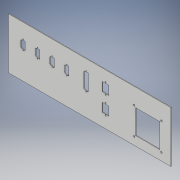
# Autodesk Inventor part: PDU_chassis
Saved by Autodesk Inventor 2017 (Build 210142000, 142)
## iProperties
Created: 2017-02-13
Part Number: PDU_chassis
Material: Generic
Document SubType Name: Modeling
Designer: Zara
Density: 1 g/cm^3
Appearance: Default
Author: Zara
Autodesk Inventor part; units mm, degrees
ref_plane "YZ Plane" through (0, 0, 0) normal (1, 0, 0) x (0, 1, 0)
ref_plane "XZ Plane" through (0, 0, 0) normal (0, 1, 0) x (-1, 0, 0)
ref_plane "XY Plane" through (0, 0, 0) normal (0, 0, 1) x (1, 0, 0)
sketch "Sketch1" plane through (0, 0, 0) normal (0, 0, 1) x (1, 0, 0)
  line L0 (-212.471, -66.7512) -> (212.471, -66.7512)
  line L1 (212.471, -66.7512) -> (212.471, 66.7512)
  line L2 (212.471, 66.7512) -> (-212.471, 66.7512)
  line L3 (-212.471, 66.7512) -> (-212.471, -66.7512)
  line L4 (-212.471, -66.7512) -> (212.471, 66.7512) construction
  line L5 (212.471, -66.7512) -> (-212.471, 66.7512) construction
  point P0 (0, 0)
  dimension "d0" = 424.942
  dimension "d1" = 133.5024
  constraints: 12 end point, 2 midpoint, 2 parallel, 1 horizontal, 1 perpendicular
  measures "d0" distance of L1.end L2.end
  measures "d1" distance of L0.end L1.end
extrude "pdu" add sketch "Sketch1" along normal blind 1.651
sketch "dsub9 sketch" plane through (0, 0, 1.651) normal (0, 0, 1) x (1, 0, 0)
  line L0 (-174.371, 28.0924) -> (-174.371, 3.0988) construction
  line L1 (-164.2108, 15.5956) -> (-184.5312, 15.5956) construction
  circle A0 centre (-174.371, 3.0988) radius 1.1303
  circle A1 centre (-174.371, 28.0924) radius 1.1303
  line L2 (-168.529, 24.7669) -> (-168.529, 6.4243)
  line L3 (-180.213, 22.9997) -> (-180.213, 8.1915)
  arc A2 (-171.1227, 4.3728) -> (-168.529, 6.4243) centre (-170.6372, 6.4243) ccw
  arc A3 (-180.213, 8.1915) -> (-178.5903, 6.14) centre (-178.1048, 8.1915) ccw
  arc A4 (-178.4938, 25.0717) -> (-180.213, 22.9997) centre (-178.1048, 22.9997) ccw
  arc A5 (-168.529, 24.0482) -> (-170.9954, 26.4795) centre (-170.6064, 24.4075) ccw
  line L4 (-170.9954, 26.4795) -> (-178.4938, 25.0717)
  line L5 (-171.1227, 4.3728) -> (-178.5903, 6.14)
  line L6 (209.423, 58.4962) -> (-209.423, 58.4962) construction
  line L7 (-209.423, 58.4962) -> (-209.423, -58.4962) construction
  line L8 (-209.423, -58.4962) -> (209.423, -58.4962) construction
  line L9 (209.423, -58.4962) -> (209.423, 58.4962) construction
  line L10 (212.471, 66.7512) -> (-212.471, 66.7512) construction
  line L11 (-212.471, -66.7512) -> (212.471, -66.7512) construction
  line L12 (-212.471, 66.7512) -> (-212.471, -66.7512) construction
  line L13 (212.471, -66.7512) -> (212.471, 66.7512) construction
  line L14 (-170.6372, 4.3161) -> (-187.2839, 4.3161) construction
  line L15 (-170.6064, 26.5157) -> (-195.0837, 26.5157) construction
  line L16 (-136.271, 28.0924) -> (-136.271, 3.0988) construction
  line L17 (-132.5064, 26.5157) -> (-156.9837, 26.5157) construction
  line L18 (-130.429, 24.7669) -> (-130.429, 6.4243)
  line L19 (-133.0227, 4.3728) -> (-140.4903, 6.14)
  circle A6 centre (-136.271, 28.0924) radius 1.1303
  circle A7 centre (-136.271, 3.0988) radius 1.1303
  line L20 (-132.5372, 4.3161) -> (-149.1839, 4.3161) construction
  line L21 (-126.1108, 15.5956) -> (-146.4312, 15.5956) construction
  arc A8 (-130.429, 24.0482) -> (-132.8954, 26.4795) centre (-132.5064, 24.4075) ccw
  line L22 (-142.113, 22.9997) -> (-142.113, 8.1915)
  line L23 (-132.8954, 26.4795) -> (-140.3938, 25.0717)
  arc A9 (-133.0227, 4.3728) -> (-130.429, 6.4243) centre (-132.5372, 6.4243) ccw
  arc A10 (-142.113, 8.1915) -> (-140.4903, 6.14) centre (-140.0048, 8.1915) ccw
  arc A11 (-140.3938, 25.0717) -> (-142.113, 22.9997) centre (-140.0048, 22.9997) ccw
  line L24 (-98.171, 28.0924) -> (-98.171, 3.0988) construction
  line L25 (-94.4064, 26.5157) -> (-118.8837, 26.5157) construction
  line L26 (-92.329, 24.7669) -> (-92.329, 6.4243)
  line L27 (-94.9227, 4.3728) -> (-102.3903, 6.14)
  circle A12 centre (-98.171, 28.0924) radius 1.1303
  circle A13 centre (-98.171, 3.0988) radius 1.1303
  line L28 (-94.4372, 4.3161) -> (-111.0839, 4.3161) construction
  line L29 (-88.0108, 15.5956) -> (-108.3312, 15.5956) construction
  arc A14 (-92.329, 24.0482) -> (-94.7954, 26.4795) centre (-94.4064, 24.4075) ccw
  line L30 (-104.013, 22.9997) -> (-104.013, 8.1915)
  line L31 (-94.7954, 26.4795) -> (-102.2938, 25.0717)
  arc A15 (-94.9227, 4.3728) -> (-92.329, 6.4243) centre (-94.4372, 6.4243) ccw
  arc A16 (-104.013, 8.1915) -> (-102.3903, 6.14) centre (-101.9048, 8.1915) ccw
  arc A17 (-102.2938, 25.0717) -> (-104.013, 22.9997) centre (-101.9048, 22.9997) ccw
  line L32 (-60.071, 28.0924) -> (-60.071, 3.0988) construction
  line L33 (-56.3064, 26.5157) -> (-80.7837, 26.5157) construction
  line L34 (-54.229, 24.7669) -> (-54.229, 6.4243)
  line L35 (-56.8227, 4.3728) -> (-64.2903, 6.14)
  circle A18 centre (-60.071, 28.0924) radius 1.1303
  circle A19 centre (-60.071, 3.0988) radius 1.1303
  line L36 (-56.3372, 4.3161) -> (-72.9839, 4.3161) construction
  line L37 (-49.9108, 15.5956) -> (-70.2312, 15.5956) construction
  arc A20 (-54.229, 24.0482) -> (-56.6954, 26.4795) centre (-56.3064, 24.4075) ccw
  line L38 (-65.913, 22.9997) -> (-65.913, 8.1915)
  line L39 (-56.6954, 26.4795) -> (-64.1938, 25.0717)
  arc A21 (-56.8227, 4.3728) -> (-54.229, 6.4243) centre (-56.3372, 6.4243) ccw
  arc A22 (-65.913, 8.1915) -> (-64.2903, 6.14) centre (-63.8048, 8.1915) ccw
  arc A23 (-64.1938, 25.0717) -> (-65.913, 22.9997) centre (-63.8048, 22.9997) ccw
  point P0 (0, 0)
  point P1 (-174.371, 15.5956)
  point P2 (-168.529, 15.5956)
  point P3 (-180.213, 15.5956)
  point P4 (-136.271, 15.5956)
  point P5 (-130.429, 15.5956)
  point P6 (-142.113, 15.5956)
  point P7 (-98.171, 15.5956)
  point P8 (-92.329, 15.5956)
  point P9 (-104.013, 15.5956)
  point P10 (-60.071, 15.5956)
  point P11 (-54.229, 15.5956)
  point P12 (-65.913, 15.5956)
  dimension "d4" = 2.2606
  dimension "d5" = 2.2606
  dimension "d6" = 24.9936
  dimension "d7" = 4.2164
  dimension "d8" = 4.2164
  dimension "d9" = 4.2164
  dimension "d10" = 4.2164
  dimension "d11" = 14.8082
  dimension "d12" = 17.9832
  dimension "d13" = 8.255
  dimension "d14" = 8.255
  dimension "d15" = 3.048
  dimension "d16" = 3.048
  dimension "d17" = 38.1
  dimension "d18" = 5.842
  dimension "d19" = 11.684
  dimension "d20" = 69.85
  dimension "d21" = 7.4985
  dimension "d24" = 38.1
  constraints: 72 end point, 44 point on circle, 24 centre point, 12 point on line, 9 tangent, 8 coincident, 5 horizontal, 4 midpoint, 3 vertical, 2 parallel, 1 perpendicular, 120 other
  measures "d4" diameter of A1
  measures "d5" diameter of A0
  measures "d6" distance of L0.start L0.end
  measures "d7" diameter of A2
  measures "d8" diameter of A3
  measures "d9" diameter of A5
  measures "d10" diameter of A4
  measures "d11" distance of A3.centre A4.centre
  measures "d12" distance of A2.centre A5.centre
  measures "d13" distance between parallel lines of L10 L6
  measures "d14" distance between parallel lines of L11 L8
  measures "d15" distance between parallel lines of L12 L7
  measures "d16" distance between parallel lines of L13 L9
  measures "d17" distance from line of L12 A0.centre
  measures "d18" distance from line of L2 A0.centre
  measures "d19" distance between parallel lines of L3 L2
  measures "d20" distance from line of L11 A0.centre
  measures "d21" horizontal distance of A4.centre A5.centre
  measures "d24" distance of A1.centre A6.centre
sketch "dsub25 sketch" plane through (0, 0, 1.651) normal (0, 0, 1) x (1, 0, 0)
  line L0 (16.129, 15.6718) -> (-34.671, 15.6718) construction
  line L1 (-9.271, 39.1922) -> (-9.271, -7.8486) construction
  circle A0 centre (-9.271, -7.8486) radius 1.1303
  circle A1 centre (-9.271, 39.1922) radius 1.1303
  line L2 (-3.429, 35.6997) -> (-3.429, -4.3561)
  line L3 (-15.113, 34.1122) -> (-15.113, -2.7686)
  arc A2 (-5.9756, -6.4182) -> (-3.429, -4.3561) centre (-5.5372, -4.3561) ccw
  arc A3 (-3.429, 35.6997) -> (-5.9756, 37.7618) centre (-5.5372, 35.6997) ccw
  arc A4 (-13.4432, 36.1743) -> (-15.113, 34.1122) centre (-13.0048, 34.1122) ccw
  arc A5 (-15.113, -2.7686) -> (-13.4432, -4.8307) centre (-13.0048, -2.7686) ccw
  line L4 (-5.9756, 37.7618) -> (-13.4432, 36.1743)
  line L5 (-5.9756, -6.4182) -> (-13.4432, -4.8307)
  line L6 (-212.471, 66.7512) -> (-212.471, -66.7512) projected
  line L7 (-212.471, -66.7512) -> (212.471, -66.7512) projected
  line L8 (-5.9756, 37.7618) -> (-23.5611, 37.7618) construction
  line L9 (-5.7893, -19.1331) -> (-33.2019, -19.1331) construction
  point P0 (0, 0)
  point P1 (-9.271, 15.6718)
  point P2 (-9.271, 15.6718)
  point P3 (-3.429, 15.6718)
  point P4 (-15.113, 15.6718)
  dimension "d31" = 2.2606
  dimension "d32" = 2.2606
  dimension "d33" = 47.0408
  dimension "d34" = 4.2164
  dimension "d35" = 4.2164
  dimension "d36" = 4.2164
  dimension "d37" = 4.2164
  dimension "d38" = 36.8808
  dimension "d39" = 40.0558
  dimension "d40" = 50.8
  dimension "d41" = 11.684
  dimension "d42" = 5.842
  dimension "d43" = 203.2
  dimension "d44" = 58.9026
  constraints: 16 end point, 8 point on circle, 8 tangent, 6 centre point, 6 midpoint, 3 vertical, 2 coincident, 2 horizontal, 2 point on line, 1 perpendicular
  measures "d31" diameter of A0
  measures "d32" diameter of A1
  measures "d33" distance of A0.centre A1.centre
  measures "d34" diameter of A2
  measures "d35" diameter of A5
  measures "d36" diameter of A4
  measures "d37" diameter of A3
  measures "d38" distance of L3.start L3.end
  measures "d39" distance of L2.start L2.end
  measures "d40" distance of L0.start L0.end
  measures "d41" distance between parallel lines of L3 L2
  measures "d42" distance from line of L2 A1.centre
  measures "d43" distance from line of L6 A1.centre
  measures "d44" distance from line of L7 A0.centre
sketch "CAT7 sketch" plane through (0, 0, 1.651) normal (0, 0, 1) x (1, 0, 0)
  line L0 (32.9565, 36.1188) -> (50.1015, 36.1188)
  line L1 (50.1015, 36.1188) -> (50.1015, 13.2588)
  line L2 (50.1015, 13.2588) -> (32.9565, 13.2588)
  line L3 (32.9565, 13.2588) -> (32.9565, 36.1188)
  line L4 (23.6736, 24.6888) -> (79.7413, 24.6888) construction
  circle A0 centre (41.529, 39.1922) radius 1.1303
  circle A1 centre (41.529, 10.1854) radius 1.1303
  line L5 (41.529, 39.1922) -> (41.529, 10.1854) construction
  line L6 (-212.471, -66.7512) -> (212.471, -66.7512) construction
  line L7 (-212.471, 66.7512) -> (-212.471, -66.7512) construction
  line L8 (32.9565, -10.922) -> (50.1015, -10.922)
  line L9 (50.1015, -10.922) -> (50.1015, -33.782)
  line L10 (50.1015, -33.782) -> (32.9565, -33.782)
  line L11 (32.9565, -33.782) -> (32.9565, -10.922)
  circle A2 centre (41.529, -7.8486) radius 1.1303
  circle A3 centre (41.529, -36.8554) radius 1.1303
  line L12 (41.529, -7.8486) -> (41.529, -36.8554) construction
  point P0 (0, 0)
  point P1 (32.9565, 24.6888)
  point P2 (41.529, 36.1188)
  point P3 (41.529, 24.6888)
  point P4 (41.529, -10.922)
  point P5 (32.9565, -22.352)
  point P6 (23.6736, -22.352)
  point P7 (41.529, -22.352)
  dimension "d47" = 22.86
  dimension "d48" = 17.145
  dimension "d49" = 2.2606
  dimension "d50" = 2.2606
  dimension "d51" = 29.0068
  dimension "d52" = 76.9366
  dimension "d53" = 254
  dimension "d56" = 47.0408
  constraints: 22 end point, 4 centre point, 4 point on line, 3 midpoint, 2 horizontal, 2 parallel, 2 vertical, 1 perpendicular, 17 other
  measures "d47" distance of L0.end L1.end
  measures "d48" distance of L1.end L2.end
  measures "d49" diameter of A0
  measures "d50" diameter of A1
  measures "d51" distance of L5.end L5.start
  measures "d52" distance from line of L6 L5.end
  measures "d53" distance from line of L7 L5.end
  measures "d56" distance of L0.start L8.start
sketch "Sketch5" plane through (0, 0, 1.651) normal (0, 0, 1) x (1, 0, 0)
  line L0 (110.109, -53.1622) -> (193.929, -53.1622) construction
  line L1 (193.929, -53.1622) -> (193.929, 30.6578) construction
  line L2 (193.929, 30.6578) -> (110.109, 30.6578) construction
  line L3 (110.109, 30.6578) -> (110.109, -53.1622) construction
  line L4 (110.109, -53.1622) -> (193.929, 30.6578) construction
  line L5 (193.929, -53.1622) -> (110.109, 30.6578) construction
  line L6 (-212.471, 66.7512) -> (-212.471, -66.7512) projected
  line L7 (-212.471, -66.7512) -> (212.471, -66.7512) projected
  line L8 (120.269, -43.0022) -> (183.769, -43.0022)
  line L9 (183.769, -43.0022) -> (183.769, 20.4978)
  line L10 (183.769, 20.4978) -> (120.269, 20.4978)
  line L11 (120.269, 20.4978) -> (120.269, -43.0022)
  line L12 (120.269, -43.0022) -> (183.769, 20.4978) construction
  line L13 (183.769, -43.0022) -> (120.269, 20.4978) construction
  line L14 (116.332, -46.9392) -> (187.706, -46.9392) construction
  line L15 (187.706, -46.9392) -> (187.706, 24.4348) construction
  line L16 (187.706, 24.4348) -> (116.332, 24.4348) construction
  line L17 (116.332, 24.4348) -> (116.332, -46.9392) construction
  line L18 (116.332, -46.9392) -> (187.706, 24.4348) construction
  line L19 (187.706, -46.9392) -> (116.332, 24.4348) construction
  circle A0 centre (116.332, 24.4348) radius 2.2479
  circle A1 centre (187.706, 24.4348) radius 2.2479
  circle A2 centre (187.706, -46.9392) radius 2.2479
  circle A3 centre (116.332, -46.9392) radius 2.2479
  line L20 (120.269, -43.0022) -> (183.769, -43.0022)
  line L21 (183.769, -43.0022) -> (183.769, 20.4978)
  line L22 (183.769, 20.4978) -> (120.269, 20.4978)
  line L23 (120.269, 20.4978) -> (120.269, -43.0022)
  line L24 (120.269, -43.0022) -> (183.769, 20.4978) construction
  line L25 (183.769, -43.0022) -> (120.269, 20.4978) construction
  point P0 (0, 0)
  point P1 (152.019, -11.2522)
  point P2 (152.019, -11.2522)
  dimension "d63" = 83.82
  dimension "d64" = 83.82
  dimension "d65" = 322.58
  dimension "d66" = 13.589
  dimension "d67" = 63.5
  dimension "d68" = 63.5
  dimension "d69" = 71.374
  dimension "d70" = 4.4958
  dimension "d71" = 4.4958
  dimension "d72" = 4.4958
  dimension "d73" = 4.4958
  constraints: 48 end point, 10 midpoint, 8 parallel, 4 centre point, 4 horizontal, 4 perpendicular, 3 coincident, 1 point on line
  measures "d63" distance of L1.end L2.end
  measures "d64" distance of L2.end L0.start
  measures "d65" distance between parallel lines of L6 L3
  measures "d66" distance between parallel lines of L0 L7
  measures "d67" distance of L8.end L9.end
  measures "d68" distance of L8.start L8.end
  measures "d69" distance of L14.start L14.end
  measures "d70" diameter of A1
  measures "d71" diameter of A0
  measures "d72" diameter of A2
  measures "d73" diameter of A3
hole "airflow holes" at (187.706, 24.4348, 1.651) at (116.332, 24.4348, 1.651) at (116.332, -46.9392, 1.651) at (187.706, -46.9392, 1.651) direction (0, 0, -1) diameter 4.4958 end through all clearance for "Flat Head Machine Screw (82)" size "#8" standard "Ansi Unified Screw Threads"
sketch "Sketch7" plane through (0, 0, 1.651) normal (0, 0, 1) x (1, 0, 0)
  line L0 (110.109, -53.1622) -> (193.929, -53.1622) construction
  line L1 (193.929, -53.1622) -> (193.929, 30.6578) construction
  line L2 (193.929, 30.6578) -> (110.109, 30.6578) construction
  line L3 (110.109, 30.6578) -> (110.109, -53.1622) construction
  line L4 (110.109, -53.1622) -> (193.929, 30.6578) construction
  line L5 (193.929, -53.1622) -> (110.109, 30.6578) construction
  line L6 (-212.471, 66.7512) -> (-212.471, -66.7512)
  line L7 (-212.471, -66.7512) -> (212.471, -66.7512)
  line L8 (120.269, -43.0022) -> (183.769, -43.0022)
  line L9 (183.769, -43.0022) -> (183.769, 20.4978)
  line L10 (183.769, 20.4978) -> (120.269, 20.4978)
  line L11 (120.269, 20.4978) -> (120.269, -43.0022)
  line L12 (120.269, -43.0022) -> (183.769, 20.4978) construction
  line L13 (183.769, -43.0022) -> (120.269, 20.4978) construction
  line L14 (116.332, -46.9392) -> (187.706, -46.9392) construction
  line L15 (187.706, -46.9392) -> (187.706, 24.4348) construction
  line L16 (187.706, 24.4348) -> (116.332, 24.4348) construction
  line L17 (116.332, 24.4348) -> (116.332, -46.9392) construction
  line L18 (116.332, -46.9392) -> (187.706, 24.4348) construction
  line L19 (187.706, -46.9392) -> (116.332, 24.4348) construction
  circle A0 centre (116.332, 24.4348) radius 2.2479
  circle A1 centre (187.706, 24.4348) radius 2.2479
  circle A2 centre (187.706, -46.9392) radius 2.2479
  circle A3 centre (116.332, -46.9392) radius 2.2479
  line L20 (120.269, -43.0022) -> (183.769, -43.0022)
  line L21 (183.769, -43.0022) -> (183.769, 20.4978)
  line L22 (183.769, 20.4978) -> (120.269, 20.4978)
  line L23 (120.269, 20.4978) -> (120.269, -43.0022)
  line L24 (120.269, -43.0022) -> (183.769, 20.4978) construction
  line L25 (183.769, -43.0022) -> (120.269, 20.4978) construction
  point P0 (0, 0)
  point P1 (0, 0)
  point P2 (152.019, -11.2522)
  point P3 (152.019, -11.2522)
  dimension "d83" = 83.82
  dimension "d84" = 83.82
  dimension "d85" = 322.58
  dimension "d86" = 13.589
  dimension "d87" = 63.5
  dimension "d88" = 63.5
  dimension "d89" = 71.374
  dimension "d90" = 4.4958
  dimension "d91" = 4.4958
  dimension "d92" = 4.4958
  dimension "d93" = 4.4958
  constraints: 52 end point, 10 midpoint, 8 parallel, 4 centre point, 4 horizontal, 4 perpendicular, 3 coincident, 1 point on line
  measures "d83" distance of L1.end L2.end
  measures "d84" distance of L2.end L0.start
  measures "d85" distance between parallel lines of L6 L3
  measures "d86" distance between parallel lines of L0 L7
  measures "d87" distance of L8.end L9.end
  measures "d88" distance of L8.start L8.end
  measures "d89" distance of L14.start L14.end
  measures "d90" diameter of A1
  measures "d91" diameter of A0
  measures "d92" diameter of A2
  measures "d93" diameter of A3
extrude "airflow cutout" cut sketch "Sketch7" against normal through all contours L11 L10 L9 L8
hole "dsub9 4-40 holes" at (-174.371, 28.0924, 1.651) at (-174.371, 3.0988, 1.651) at (-136.271, 3.0988, 1.651) at (-136.271, 28.0924, 1.651) at (-98.171, 28.0924, 1.651) at (-98.171, 3.0988, 1.651) at (-60.071, 28.0924, 1.651) at (-60.071, 3.0988, 1.651) direction (0, 0, -1) diameter 2.159 depth 8.8646 tip angle 118
extrude "dsub9 cutouts" cut sketch "dsub9 sketch" against normal through all contours L2 A2 L5 A3 L3 A4 L4 A5 | L18 A9 L19 A10 L22 A11 L23 A8 | L26 A15 L27 A16 L30 A17 L31 A14 | L34 A21 L35 A22 L38 A23 L39 A20
hole "CAT7 holes" at (41.529, 39.1922, 1.651) at (41.529, 10.1854, 1.651) at (41.529, -7.8486, 1.651) at (41.529, -36.8554, 1.651) direction (0, 0, -1) diameter 2.9464 end through all
extrude "CAT7 cutout" cut sketch "CAT7 sketch" against normal through all contours L0 L1 L2 L3 | L8 L9 L10 L11
hole "dsub25 4-40 holes" at (-9.271, 39.1922, 1.651) at (-9.271, -7.8486, 1.651) direction (0, 0, -1) diameter 2.159 end through all
extrude "dsub25 cutout" cut sketch "dsub25 sketch" against normal through all contours L2 A2 L5 A5 L3 A4 L4 A3
body "Solid1"
